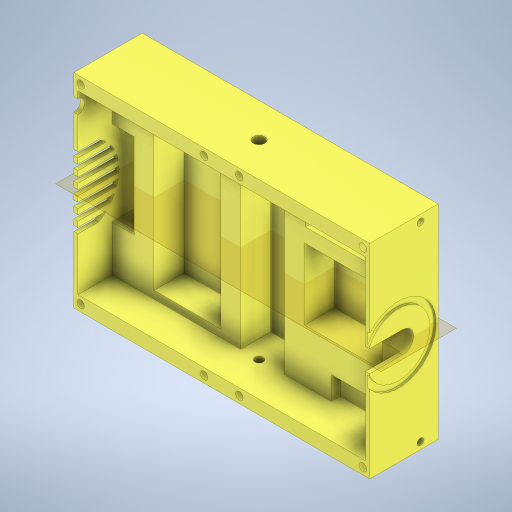
# Autodesk Inventor part: caseLowerPortion
Saved by Autodesk Inventor 2023 (Build 270158030, 158C)
## iProperties
Created: 2021-08-20
Part Number: caseLowerPortion
Material: PC/ABS Plastic
Document SubType Name: Modeling
Designer: robst
Density: 0.357273 g/cm^3
Appearance: Smooth - Yellow
Author: robst
Autodesk Inventor part; units mm, degrees
ref_plane "YZ Plane" through (0, 0, 0) normal (1, 0, 0) x (0, 1, 0)
ref_plane "XY Plane" through (0, 0, 0) normal (0, 0, 1) x (1, 0, 0)
sketch "Sketch1" plane through (0, 0, 0) normal (0, 0, 1) x (1, 0, 0)
  line L0 (-108.1, -74.5) -> (108.1, -74.5)
  line L1 (108.1, -74.5) -> (108.1, 74.5)
  line L2 (108.1, 74.5) -> (-108.1, 74.5)
  line L3 (-108.1, 74.5) -> (-108.1, -74.5)
  line L4 (-108.1, -74.5) -> (108.1, 74.5) construction
  line L5 (108.1, -74.5) -> (-108.1, 74.5) construction
  point P0 (0, 0)
  dimension "d0" = 216.2
  dimension "d1" = 149
  constraints: 12 end point, 2 midpoint, 2 parallel, 1 horizontal, 1 perpendicular
  measures "d0" distance of L0.start L0.end
  measures "d1" distance of L1.end L0.end
extrude "MainInnerBodyExtrusion" add sketch "Sketch1" against normal blind 50
sketch "Sketch3" plane through (0, 0, 0) normal (0, 0, 1) x (1, 0, 0)
  line L0 (35.4, -26) -> (92.4, -26)
  line L1 (92.4, -26) -> (92.4, 26)
  line L2 (92.4, 26) -> (35.4, 26)
  line L3 (35.4, 26) -> (35.4, -26)
  line L4 (35.4, -26) -> (92.4, 26) construction
  line L5 (92.4, -26) -> (35.4, 26) construction
  line L6 (108.1, -74.5) -> (108.1, 74.5) projected
  line L7 (0, 0) -> (108.1, 0) construction
  line L8 (-108.1, -74.5) -> (-108.1, 74.5) construction
  line L9 (-108.1, 74.5) -> (-108.1, -74.5) projected
  point P0 (63.9, 0)
  point P1 (63.9, 0)
  dimension "d5" = 15.7
  dimension "d6" = 52
  dimension "d7" = 57
  constraints: 14 end point, 4 midpoint, 2 parallel, 1 horizontal, 1 perpendicular, 1 point on line
  measures "d5" distance between parallel lines of L1 L6
  measures "d6" distance of L0.end L1.end
  measures "d7" distance of L1.end L2.end
extrude "HoleForCamerabase" cut sketch "Sketch3" against normal blind 47
sketch "Sketch4" plane through (0, 0, 0) normal (0, 0, 1) x (1, 0, 0)
  line L0 (0, 0) -> (-108.1, 0) construction
  line L1 (-108.1, -74.5) -> (-108.1, 74.5) construction
  line L2 (-105.1, -31) -> (-89.1, -31)
  line L3 (-89.1, -31) -> (-89.1, 31)
  line L4 (-89.1, 31) -> (-105.1, 31)
  line L5 (-105.1, 31) -> (-105.1, -31)
  line L6 (-105.1, -31) -> (-89.1, 31) construction
  line L7 (-89.1, -31) -> (-105.1, 31) construction
  point P0 (-97.1, 0)
  dimension "d13" = 16
  dimension "d14" = 62
  dimension "d15" = 3
  constraints: 14 end point, 3 midpoint, 2 parallel, 1 perpendicular, 1 point on line
  measures "d13" distance of L2.start L2.end
  measures "d14" distance of L3.end L2.end
  measures "d15" distance between parallel lines of L1 L5
extrude "HoleForFan" cut sketch "Sketch4" against normal blind 47
sketch "Sketch6" plane through (0, 0, 0) normal (0, 0, 1) x (1, 0, 0)
  line L0 (-108.1, -74.5) -> (-108.1, 74.5) construction
  line L1 (-108.1, 0) -> (108.1, 0) construction
  line L2 (108.1, 74.5) -> (108.1, -74.5) construction
  line L3 (-11.1, -64.5) -> (20.9, -64.5)
  line L4 (20.9, -64.5) -> (20.9, 64.5)
  line L5 (20.9, 64.5) -> (-11.1, 64.5)
  line L6 (-11.1, 64.5) -> (-11.1, -64.5)
  line L7 (-11.1, -64.5) -> (20.9, 64.5) construction
  line L8 (20.9, -64.5) -> (-11.1, 64.5) construction
  line L9 (35.4, -26) -> (35.4, 26) projected
  point P0 (0, 0)
  point P1 (4.9, 0)
  dimension "d20" = 32
  dimension "d21" = 129
  dimension "d88" = 14.5
  constraints: 14 end point, 4 midpoint, 3 parallel, 1 perpendicular, 1 point on line
  measures "d20" distance of L3.start L3.end
  measures "d21" distance of L4.end L3.end
  measures "d88" distance between parallel lines of L4 L9
extrude "HoleForPi" cut sketch "Sketch6" against normal blind 47
sketch "Sketch7" plane through (0, 0, 0) normal (0, 0, 1) x (1, 0, 0)
  line L0 (0, 0) -> (-108.1, 0) construction
  line L1 (-108.1, 74.5) -> (-108.1, -74.5) construction
  line L2 (-74.6, -59) -> (-25.6, -59)
  line L3 (-25.6, -59) -> (-25.6, 59)
  line L4 (-25.6, 59) -> (-74.6, 59)
  line L5 (-74.6, 59) -> (-74.6, -59)
  line L6 (-74.6, -59) -> (-25.6, 59) construction
  line L7 (-25.6, -59) -> (-74.6, 59) construction
  line L8 (-11.1, -64.5) -> (-11.1, 64.5) projected
  line L9 (-89.1, 31) -> (-89.1, -31) construction
  point P0 (-50.1, 0)
  dimension "d25" = 14.5
  dimension "d26" = 49
  dimension "d27" = 118
  constraints: 14 end point, 3 midpoint, 2 parallel, 1 perpendicular, 1 point on line
  measures "d25" distance between parallel lines of L3 L8
  measures "d26" distance of L2.start L2.end
  measures "d27" distance of L4.end L2.start
extrude "HoleForPoeAdapter" cut sketch "Sketch7" against normal blind 47
sketch "Sketch10" plane through (0, 0, 0) normal (0, 0, 1) x (1, 0, 0)
  line L0 (36.1, 36.5) -> (105.1, 36.5)
  line L1 (105.1, 36.5) -> (105.1, 64.5)
  line L2 (105.1, 64.5) -> (36.1, 64.5)
  line L3 (36.1, 64.5) -> (36.1, 36.5)
  line L4 (36.1, 36.5) -> (105.1, 64.5) construction
  line L5 (105.1, 36.5) -> (36.1, 64.5) construction
  line L6 (108.1, 74.5) -> (-108.1, 74.5) projected
  line L7 (108.1, -74.5) -> (108.1, 74.5) projected
  point P0 (0, 0)
  point P1 (70.6, 50.5)
  point P2 (94.85, 8.5)
  point P3 (105.1, 50.5)
  dimension "d36" = 69
  dimension "d37" = 28
  dimension "d85" = 3
  constraints: 12 end point, 3 midpoint, 2 parallel, 1 horizontal, 1 perpendicular, 1 other
  measures "d36" distance of L1.end L2.end
  measures "d37" distance of L0.end L1.end
extrude "HoleForThermister" cut sketch "Sketch10" against normal blind 47
sketch "Sketch11" plane through (0, 0, 0) normal (0, 0, 1) x (1, 0, 0)
  line L0 (55.1, -64.5) -> (105.1, -64.5)
  line L1 (105.1, -64.5) -> (105.1, -47.5)
  line L2 (105.1, -47.5) -> (55.1, -47.5)
  line L3 (55.1, -47.5) -> (55.1, -64.5)
  line L4 (55.1, -64.5) -> (105.1, -47.5) construction
  line L5 (105.1, -64.5) -> (55.1, -47.5) construction
  line L6 (108.1, -74.5) -> (108.1, 74.5) projected
  line L7 (-108.1, -74.5) -> (108.1, -74.5) projected
  line L8 (92.4, -26) -> (35.4, -26) projected
  line L9 (20.9, 64.5) -> (20.9, -64.5) projected
  point P0 (0, 0)
  point P1 (80.1, -56)
  point P2 (94.85, -8.5)
  point P3 (80.1, -47.5)
  point P4 (55.1, -56)
  point P5 (108.1, 74.5)
  dimension "d42" = 50
  dimension "d43" = 17
  dimension "d86" = 3
  dimension "d87" = 10
  constraints: 12 end point, 4 midpoint, 2 parallel, 1 horizontal, 1 perpendicular, 1 other
  measures "d42" distance of L0.start L0.end
  measures "d43" distance of L0.end L1.end
  measures "d87" distance between parallel lines of L7 L0
extrude "HoleForSensor" cut sketch "Sketch11" against normal blind 31.5
sketch "Sketch15" plane through (-108.1, -74.5, 0) normal (-1, 0, 0) x (0, 0, 1)
  line L0 (0, 149) -> (0, 0) projected
  line L1 (0, 149) -> (-50, 149) projected
  line L2 (-50, 0) -> (-50, 149) projected
  line L3 (0, 0) -> (-50, 0) projected
  line L4 (0, 0) -> (0, 149) projected
  line L5 (0, 100.5) -> (0, 48.5) projected
  line L6 (0, 74.5) -> (-30, 74.5) construction
  line L7 (0, 76.5) -> (-29.9333, 76.5)
  line L8 (0, 84.5) -> (-28.2843, 84.5)
  line L9 (0, 80.5) -> (-29.3939, 80.5)
  line L10 (0, 76.5) -> (0, 74.5)
  line L11 (0, 88.5) -> (-26.533, 88.5)
  line L12 (0, 92.5) -> (-24, 92.5)
  line L13 (-20.3961, 96.5) -> (0, 96.5)
  line L14 (-14.9666, 100.5) -> (0, 100.5)
  line L15 (0, 84.5) -> (0, 80.5)
  line L16 (0, 100.5) -> (0, 96.5)
  line L17 (0, 92.5) -> (0, 88.5)
  line L18 (0, 72.5) -> (-29.9333, 72.5)
  line L19 (0, 64.5) -> (-28.2843, 64.5)
  line L20 (0, 68.5) -> (-29.3939, 68.5)
  line L21 (0, 72.5) -> (0, 74.5)
  line L22 (0, 60.5) -> (-26.533, 60.5)
  line L23 (0, 56.5) -> (-24, 56.5)
  line L24 (-20.3961, 52.5) -> (0, 52.5)
  line L25 (-14.9666, 48.5) -> (0, 48.5)
  line L26 (0, 64.5) -> (0, 68.5)
  line L27 (0, 56.5) -> (0, 60.5)
  line L28 (0, 48.5) -> (0, 52.5)
  line L29 (0, 72.5) -> (0, 76.5)
  line L30 (0, 80.5) -> (0, 84.5)
  line L31 (0, 88.5) -> (0, 92.5)
  line L32 (0, 96.5) -> (0, 149)
  arc A0 (-28.2843, 84.5) -> (-29.3939, 80.5) centre (0, 74.5) ccw
  arc A1 (-14.9666, 100.5) -> (-20.3961, 96.5) centre (0, 74.5) ccw
  arc A2 (-24, 92.5) -> (-26.533, 88.5) centre (0, 74.5) ccw
  arc A3 (-29.9333, 76.5) -> (-29.9333, 72.5) centre (0, 74.5) ccw
  arc A4 (-29.3939, 68.5) -> (-28.2843, 64.5) centre (0, 74.5) ccw
  arc A5 (-26.533, 60.5) -> (-24, 56.5) centre (0, 74.5) ccw
  arc A6 (-20.3961, 52.5) -> (-14.9666, 48.5) centre (0, 74.5) ccw
  point P0 (0, 74.5)
  point P1 (0, 82)
  point P2 (0, 67.0167)
  point P3 (0, 4.25)
  point P4 (-10.198, 96.5)
  point P5 (0, 48.5)
  point P6 (0, 52.5)
  point P7 (0, 56.5)
  point P8 (0, 60.5)
  point P9 (0, 64.5)
  point P10 (0, 68.5)
  point P11 (0, 72.5)
  point P12 (0, 80.5)
  point P13 (0, 84.5)
  point P14 (0, 88.5)
  point P15 (0, 92.5)
  point P16 (0, 96.5)
  point P17 (0, 100.5)
  dimension "d69" = 2
  dimension "d71" = 4
  dimension "d72" = 4
  dimension "d73" = 4
  dimension "d75" = 4
  dimension "d142" = 30
  constraints: 54 end point, 15 point on circle, 15 symmetric about line, 7 centre point, 3 parallel, 3 perpendicular, 2 horizontal, 1 coincident, 1 midpoint, 1 other
  measures "d69" distance between parallel lines of L7 L6
  measures "d71" distance between parallel lines of L8 L9
  measures "d72" distance between parallel lines of L11 L8
  measures "d73" distance between parallel lines of L12 L11
  measures "d75" distance between parallel lines of L13 L14
  measures "d142" radius of A2
extrude "SlotsForRearFan" cut sketch "Sketch15" against normal up to surface (3 mm away) contours L0 L13 A1 L14 | L0 L11 A2 L12 | L25 A6 L24 L0 | L0 L9 A0 L8 | L23 A5 L22 L0 | L0 L18 A3 L7 | L19 A4 L20 L0
sketch "Sketch16" plane through (0, 0, -47) normal (0, 0, 1) x (1, 0, 0)
  line L0 (92.4, 26) -> (92.4, -26) projected
  line L1 (76.9, 10.765) -> (76.9, -11.235) construction
  line L2 (75.4, 10.765) -> (75.4, -11.235)
  line L3 (72.4, -11.235) -> (72.4, 10.765)
  line L4 (69.4, 8.7746) -> (69.4, -9.2446)
  line L5 (66.4, 3.5785) -> (66.4, -4.0485)
  line L6 (78.4, 10.765) -> (78.4, -11.235)
  line L7 (81.4, -11.235) -> (81.4, 10.765)
  line L8 (84.4, 8.7746) -> (84.4, -9.2446)
  line L9 (87.4, 3.5785) -> (87.4, -4.0485)
  line L10 (70.5491, 10.765) -> (72.4, 10.765)
  line L11 (72.4, -11.235) -> (70.5491, -11.235)
  line L12 (70.5491, -11.235) -> (69.4, -9.2446)
  line L13 (66.4, -4.0485) -> (64.1983, -0.235)
  line L14 (64.1983, -0.235) -> (66.4, 3.5785)
  line L15 (69.4, 8.7746) -> (70.5491, 10.765)
  line L16 (75.4, 10.765) -> (78.4, 10.765)
  line L17 (81.4, 10.765) -> (83.2509, 10.765)
  line L18 (83.2509, -11.235) -> (81.4, -11.235)
  line L19 (78.4, -11.235) -> (75.4, -11.235)
  line L20 (89.6017, -0.235) -> (87.4, -4.0485)
  line L21 (84.4, -9.2446) -> (83.2509, -11.235)
  line L22 (83.2509, 10.765) -> (84.4, 8.7746)
  line L23 (87.4, 3.5785) -> (89.6017, -0.235)
  point P0 (0, 0)
  point P1 (76.9, -0.235)
  point P2 (66.4, -0.235)
  dimension "d78" = 15.5
  dimension "d89" = 1.5
  dimension "d90" = 3
  dimension "d91" = 3
  dimension "d92" = 3
  constraints: 46 end point, 8 symmetric about line, 6 perpendicular, 3 horizontal, 3 midpoint, 2 vertical, 7 other
  measures "d78" distance from line of point (76.9, -0.235) L0
  measures "d89" distance between parallel lines of L2 L1
  measures "d90" distance between parallel lines of L3 L2
  measures "d91" distance between parallel lines of L4 L3
  measures "d92" distance from line of point (66.4, -0.235) L4
extrude "VentForCamera" cut sketch "Sketch16" against normal through all
sketch "Sketch18" plane through (108.1, -74.5, 0) normal (1, 0, 0) x (0, 0, -1)
  line L0 (0, 74.5) -> (29.6767, 74.5) construction
  arc A0 (24, 66.5) -> (24, 82.5) centre (24, 74.5) ccw
  line L1 (0, 0) -> (0, 149) projected
  line L2 (24, 82.5) -> (0, 82.5)
  line L3 (24, 66.5) -> (0, 66.5)
  line L4 (0, 82.5) -> (0, 66.5)
  point P0 (0, 74.5)
  dimension "d97" = 16
  dimension "d137" = 24
  constraints: 8 end point, 3 point on line, 2 perpendicular, 2 point on circle, 2 tangent, 1 centre point, 1 collinear, 1 horizontal, 1 midpoint
  measures "d97" diameter of A0
  measures "d137" distance of point (0, 74.5) A0.centre
extrude "HoleForLens" cut sketch "Sketch18" against normal up to surface (15.7 mm away)
sketch "Sketch23" plane through (0, 0, 0) normal (0, 0, 1) x (1, 0, 0)
  line L0 (-103.1, -69.5) -> (103.1, -69.5) construction
  line L1 (103.1, -69.5) -> (103.1, 69.5) construction
  line L2 (103.1, 69.5) -> (-103.1, 69.5) construction
  line L3 (-103.1, 69.5) -> (-103.1, -69.5) construction
  line L4 (-103.1, -69.5) -> (103.1, 69.5) construction
  line L5 (103.1, -69.5) -> (-103.1, 69.5) construction
  line L6 (108.1, -74.5) -> (108.1, -8) projected
  line L7 (108.1, 74.5) -> (-108.1, 74.5) projected
  line L8 (-108.1, -26) -> (-108.1, -74.5) projected
  line L9 (-108.1, 74.5) -> (-108.1, 26) projected
  line L10 (108.1, 8) -> (108.1, 74.5) projected
  point P0 (0, 0)
  point P1 (12.85, -69.5)
  point P2 (-12.85, -69.5)
  point P3 (-12.85, 69.5)
  point P4 (12.85, 69.5)
  dimension "d106" = 5
  dimension "d108" = 5
  dimension "d222" = 95.25
  dimension "d223" = 95.25
  dimension "d224" = 95.25
  dimension "d225" = 95.25
  constraints: 12 end point, 4 coincident, 4 point on line, 2 midpoint, 2 parallel, 1 horizontal, 1 perpendicular
  measures "d106" distance between parallel lines of L1 L6
  measures "d108" distance between parallel lines of L2 L7
  measures "d222" distance from line of point (12.85, -69.5) L6
  measures "d223" distance from line of point (-12.85, -69.5) L8
  measures "d224" distance from line of point (-12.85, 69.5) L9
  measures "d225" distance from line of point (12.85, 69.5) L10
hole "Hole for 6-32 Insert" at (-103.1, 69.5, 0) at (103.1, 69.5, 0) at (103.1, -69.5, 0) at (-103.1, -69.5, 0) at (-12.85, -69.5, 0) at (12.85, -69.5, 0) at (-12.85, 69.5, 0) at (12.85, 69.5, 0) direction (0, 0, -1) diameter 4.7 depth 7.2 tip angle 118 counterbore diameter 5.54 counterbore depth 5.55
hole "Screw hole for 6-32 screw" at (-103.1, -69.5, 0) at (103.1, -69.5, 0) at (103.1, 69.5, 0) at (-103.1, 69.5, 0) direction (0, 0, -1) diameter 3.797 depth 15 tip angle 118 clearance for "Hex Machine Screw" size "#6" standard "Ansi Unified Screw Threads"
sketch "Sketch24" plane through (-108.1, -74.5, 0) normal (0, -1, 0) x (1, 0, 0)
  line L0 (0, -50) -> (216.2, -50) construction
  line L1 (216.2, 0) -> (200.5, 0) construction
  line L2 (0, 0) -> (0, -50) projected
  point P0 (108.1, 0)
  point P1 (110.35, -25)
  dimension "d143" = 25
  dimension "d147" = 110.35
  constraints: 2 other
  measures "d143" distance from line of point (110.35, -25) L0
  measures "d147" distance from line of point (110.35, -25) L2
hole "Side hole for 1-4 20 insert" at (2.25, -74.5, -25) direction (0, 1, 0) diameter 7.666 depth 9.53 tip angle 118 counterbore diameter 8.406 counterbore depth 7.41 clearance for "Hex Machine Screw" size "1/4" standard "Ansi Unified Screw Threads"
mirror "Mirror for side insert" about plane through (0, 0, 0) normal (0, 1, 0) of "Side hole for 1-4 20 insert"
sketch "Sketch25" plane through (0, 0, 0) normal (0, 0, 1) x (1, 0, 0)
  line L0 (108.1, 74.5) -> (-108.1, 74.5) projected
  line L1 (-108.1, 74.5) -> (-108.1, 26) projected
  line L2 (-108.1, -74.5) -> (108.1, -74.5) projected
  line L3 (78.4, -11.235) -> (75.4, -11.235) projected
  line L4 (75.4, -11.235) -> (75.4, 10.765) projected
  line L5 (75.4, 10.765) -> (78.4, 10.765) projected
  line L6 (78.4, 10.765) -> (78.4, -11.235) projected
  line L7 (70.5491, 10.765) -> (72.4, 10.765) projected
  line L8 (72.4, 10.765) -> (72.4, -11.235) projected
  line L9 (72.4, -11.235) -> (70.5491, -11.235) projected
  line L10 (70.5491, -11.235) -> (69.4, -9.2446) projected
  line L11 (69.4, -9.2446) -> (69.4, 8.7746) projected
  line L12 (69.4, 8.7746) -> (70.5491, 10.765) projected
  line L13 (84.4, 8.7746) -> (84.4, -9.2446) projected
  line L14 (84.4, -9.2446) -> (83.2509, -11.235) projected
  line L15 (83.2509, -11.235) -> (81.4, -11.235) projected
  line L16 (81.4, -11.235) -> (81.4, 10.765) projected
  line L17 (81.4, 10.765) -> (83.2509, 10.765) projected
  line L18 (83.2509, 10.765) -> (84.4, 8.7746) projected
  line L19 (66.4, 3.5785) -> (66.4, -4.0485) projected
  line L20 (66.4, -4.0485) -> (64.1983, -0.235) projected
  line L21 (64.1983, -0.235) -> (66.4, 3.5785) projected
  line L22 (89.6017, -0.235) -> (87.4, -4.0485) projected
  line L23 (87.4, -4.0485) -> (87.4, 3.5785) projected
  line L24 (87.4, 3.5785) -> (89.6017, -0.235) projected
  line L25 (92.4, 26) -> (92.4, -26) projected
  line L26 (35.4, 26) -> (92.4, 26) projected
  line L27 (35.4, -26) -> (35.4, 26) projected
  line L28 (92.4, -26) -> (35.4, -26) projected
  line L29 (108.1, -74.5) -> (108.1, -8) projected
  line L30 (108.1, 8) -> (108.1, 74.5) projected
  line L31 (-105.1, -64.5) -> (105.1, -64.5)
  line L32 (105.1, -64.5) -> (105.1, 64.5)
  line L33 (105.1, 64.5) -> (-105.1, 64.5)
  line L34 (-105.1, 64.5) -> (-105.1, -64.5)
  line L35 (-105.1, -64.5) -> (105.1, 64.5) construction
  line L36 (105.1, -64.5) -> (-105.1, 64.5) construction
  line L37 (-25.6, 59) -> (-25.6, -59) projected
  point P0 (0, 0)
  dimension "d138" = 10
  dimension "d139" = 3
  constraints: 12 end point, 2 midpoint, 2 parallel, 2 perpendicular
  measures "d138" distance between parallel lines of L2 L31
  measures "d139" distance between parallel lines of L1 L34
extrude "Extrusion18" cut sketch "Sketch25" against normal blind 25 contours L34 L33 L32 L31
sketch "Sketch26" plane through (-108.1, -74.5, -50) normal (-1, 0, 0) x (0, 0, 1)
  arc A0 (50, 124) -> (50, 134) centre (50, 129) ccw
  circle A1 centre (50, 129) radius 5
  point P0 (50, 74.5)
  point P1 (50, 124)
  constraints: 2 centre point, 2 point on circle, 1 coincident, 1 concentric, 4 other
extrude "Extrusion19" cut sketch "Sketch26" against normal up to surface (3 mm away)
sketch "Sketch30" plane through (108.1, -74.5, -50) normal (1, 0, 0) x (0, 0, -1)
  circle A0 centre (-29, 74.5) radius 27.5
  line L0 (0, 149) -> (0, 0) projected
  circle A1 centre (-29, 74.5) radius 23
  line L1 (-50, 0) -> (-50, 66.5) projected
  point P0 (-50, 74.5)
  dimension "d162" = 55
  dimension "d163" = 29
  dimension "d164" = 46
  dimension "d165" = 21
  constraints: 2 centre point, 1 coincident
  measures "d162" diameter of A0
  measures "d163" distance from line of L0 A0.centre
  measures "d164" diameter of A1
  measures "d165" distance from line of L1 A0.centre
extrude "Extrusion20" cut sketch "Sketch30" against normal blind 1.5
sketch "Sketch35" plane through (108.1, -74.5, -50) normal (1, 0, 0) x (0, 0, -1)
  circle A0 centre (-13, 5) radius 2.4257
  circle A1 centre (-13, 144) radius 2.4257
  line L0 (-50, 0) -> (0, 0) projected
  line L1 (-50, 149) -> (0, 149) projected
  line L2 (-3, 139) -> (-3, 10) projected
  point P0 (-50, 74.5)
  dimension "d215" = 4.8514
  dimension "d216" = 5
  dimension "d217" = 5
  dimension "d218" = 10
  dimension "d219" = 10
  constraints: 2 centre point, 1 equal radius
  measures "d215" diameter of A1
  measures "d216" distance from line of A0.centre L0
  measures "d217" distance from line of A1.centre L1
  measures "d218" distance from line of A0.centre L2
  measures "d219" distance from line of A1.centre L2
extrude "Extrusion21" cut sketch "Sketch35" against normal blind 9.525
equation "\"d0\" = newCaseLength"
equation "\"d1\" = caseWidth"
equation "\"d2\" = caseDepth"
equation "\"d5\" = lensLength"
equation "\"d6\" = cameraWidth"
equation "\"d7\" = cameraLength"
equation "\"d8\" = maxComponentDepth"
equation "\"d13\" = fanDepth"
equation "\"d14\" = fanWidth"
equation "\"d15\" = rearWallThickness"
equation "\"d16\" = maxComponentDepth"
equation "\"d20\" = piCaseDepth"
equation "\"d21\" = piCaseLength"
equation "\"d88\" = minDelta"
equation "\"d22\" = maxComponentDepth"
equation "\"d25\" = minDelta"
equation "\"d26\" = poeWidth"
equation "\"d27\" = poeLength"
equation "\"d28\" = maxComponentDepth"
equation "\"d36\" = thermisterLength"
equation "\"d37\" = thermisterWidth"
equation "\"d85\" = frontWallThickness"
equation "\"d38\" = maxComponentDepth"
equation "\"d42\" = sensorLength"
equation "\"d43\" = sensorWidth"
equation "\"d86\" = frontWallThickness"
equation "\"d87\" = outsideWallThickness"
equation "\"d46\" = cutoutDepth"
equation "\"outsideWallThickness\" = 10"
equation "\"caseWidth\" = piCaseLength + 2 * outsideWallThickness"
equation "\"oneHalfCaseDepth\" = piCaseWidth"
equation "\"caseLength\" = 189.7"
equation "\"lensLength\" = 15.7"
equation "\"piCaseWidth\" = 63"
equation "\"piCaseDepth\" = 32"
equation "\"poeDepth\" = 38"
equation "\"piEthernetCableReliefLength\" = 35"
equation "\"poeEthernetCableReliefLength\" = 35"
equation "\"thermisterDepth\" = 18"
equation "\"sensorDepth\" = 11"
equation "\"cutoutDepth\" = 0.5 * piCaseWidth"
equation "\"thickenDistance\" = 1"
equation "\"bottomOfCaseWallThickness\" = 3"
equation "\"rearWallThickness\" = 3"
equation "\"maxComponentDepth\" = extraCutoutDepth + 0.5 * piCaseWidth"
equation "\"caseDepth\" = maxComponentDepth + bottomOfCaseWallThickness"
equation "\"minDelta\" = 14.5"
equation "\"fanCutoutDepth\" = 0.5 * fanLength + extraCutoutDepth + thickenDistance"
equation "\"newCaseLength\" = cameraLength + piCaseDepth + fanDepth + poeWidth + rearWallThickness + 3 * minDelta + lensLength"
equation "\"frontWallThickness\" = 3"
equation "\"d95\" = lensDiameter"
equation "\"extraCutoutDepth\" = 15.5"
equation "\"cameraWidth\" = 52"
equation "\"cameraLength\" = 57"
equation "\"fanDepth\" = 16"
equation "\"fanWidth\" = 62"
equation "\"piCaseLength\" = 129"
equation "\"poeWidth\" = 49"
equation "\"poeLength\" = 118"
equation "\"thermisterLength\" = 69"
equation "\"thermisterWidth\" = 28"
equation "\"sensorLength\" = 50"
equation "\"sensorWidth\" = 17"
equation "\"fanLength\" = 60"
equation "\"lensDiameter\" = 15"
body "Solid1"
